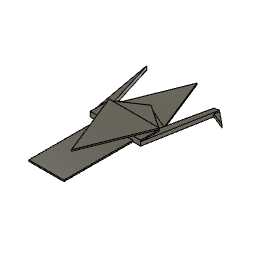
OrigamiBookmark v4 (Autodesk Fusion 360 design; units mm, degrees)
Autodesk Fusion 360 part; units mm, degrees
note: some values were not read from the file. Chosen so that the rebuilt part matches the saved one: which bodies a step acts on. Set by a fixed rule: which sketch regions a step uses.
sketch "Sketch1" plane through (0, 0, 0) normal (0, 0, 1) x (1, 0, 0)
  line L0 (18.6165, 3.413) -> (0.0203, 50.0507)
  line L1 (-20, 0) -> (0, -50)
  line L2 (20, 0) -> (0, -50)
  line L3 (-20, -15) -> (-14, -15)
  line L4 (-20, -15) -> (-20, -0.0774)
  line L5 (-20, -15) -> (-30, 40)
  line L6 (-20, -10) -> (-20, -20) construction
  line L7 (20, -15) -> (14, -15)
  line L8 (20, -15) -> (20, 0)
  line L9 (20, -15) -> (29.6805, 38.2428)
  line L10 (28.9908, 34.4493) -> (40, 30)
  line L11 (29.2258, 38.7285) -> (40, 30)
  line L12 (-17.9674, 1.3624) -> (-30, 40)
  line L13 (29.2258, 38.7285) -> (26.0078, 37.4454)
  line L14 (-18.606, 3.413) -> (18.6165, 3.413) construction
  line L15 (18.1455, 1.2446) -> (26.0078, 37.4454)
  line L16 (29.6805, 38.2428) -> (26.0078, 37.4454)
  line L17 (29.6805, 38.2428) -> (29.7947, 38.2676)
  line L18 (0.0129, 13.4141) -> (-20, 0)
  line L19 (0.0129, 13.4141) -> (20, 0)
  line L20 (0.0129, 13.4141) -> (-17.679, 5.7341)
  line L21 (0, 0) -> (0.219, 1.2047)
  line L22 (0.0203, 50.0507) -> (0.0052, 3.413) construction
  line L23 (0.0129, 13.4141) -> (17.6955, 5.7226)
  line L24 (-18.606, 3.413) -> (0.0203, 50.0507)
  line L25 (-20, 0) -> (-20, -0.0774)
  line L26 (-20, 0) -> (20, 0)
  line L27 (-14, -15) -> (-14, -115)
  line L28 (14, -15) -> (14, -115)
  line L29 (-14, -15) -> (14, -15)
  line L30 (-14, -115) -> (-14, -140)
  line L31 (14, -115) -> (14, -140)
  line L32 (14, -140) -> (-14, -140)
  dimension "d13" = 100
  dimension "d14" = 100
  constraint coincident L1 L3.end
  constraint horizontal L3
  constraint perpendicular L3 L4
  constraint perpendicular L3 L6
  constraint midpoint L3.start L6
  constraint coincident L2 L7.end
  constraint perpendicular L7 L8
  constraint coincident L9 L10.start
  constraint perpendicular L0 L13
  constraint horizontal L14
  constraint coincident L11 L17.end
  constraint parallel L16 L17
  constraint coincident L21.start origin
  constraint parallel L9 L21
  constraint midpoint L14 L22.end
  constraint coincident L0 L23.end
  constraint coincident L19 L15.start
  constraint coincident L0.start L15
  constraint coincident L18 L12.start
  constraint coincident L14.start L12
  constraint parallel L4 L25
  constraint perpendicular L8 L26
  constraint perpendicular L3 L27
  constraint perpendicular L7 L28
  constraint perpendicular L28 L29
  constraint perpendicular L30 L32
  measures "d13" distance of L3.end L27.end
  measures "d14" distance of L7.end L28.end
extrude "Extrude1" add sketch "Sketch1" along normal blind 1 contours L0 L20 L23 L24 makes body 1
extrude "Extrude2" add sketch "Sketch1" along normal blind 2 separate body contours L0 L15 L19 L23 | L11 L13 L16 L17 | L12 L18 L20 L24 makes body 2 at (-5.9806, 9.3969, 0.6667) makes body 2 at (6.0571, 9.3576, 0.6667) makes body 3 at (27.2701, 37.7194, 1.3333)
extrude "Extrude3" add sketch "Sketch1" along normal blind 3 contours L8 L9 L15 L16 L19 | L4 L5 L12 L18 L25 bodies 3 2
extrude "Extrude4" add sketch "Sketch1" along normal blind 2 separate body contours L9 L10 L11 L17 makes body 4
extrude "Extrude5" add sketch "Sketch1" along normal blind 4 contours L18 L19 L26 | L2 L7 L8 | L1 L3 L4 L25 bodies 3 4 1
extrude "Extrude6" add sketch "Sketch1" along normal blind 5 contours L1 L2 L26 L29 | L1 L2 L29 bodies 3
sketch "Sketch2" plane through (0, 0, 0) normal (0, 0, 1) x (1, 0, 0)
sketch "Sketch3" plane through (0, 0, 0) normal (0, 0, 1) x (1, 0, 0)
  line L0 (-14, -15) -> (-14, -115)
  line L1 (-14, -15) -> (14, -15)
  line L2 (14, -15) -> (14, -115)
  line L3 (-14, -115) -> (14, -115)
  line L4 (-14, -115) -> (14, -115)
  line L5 (14, -15) -> (-14, -15)
  line L6 (-14, -115) -> (-14, -15)
  line L7 (-14, -115) -> (-14, -140)
  line L8 (14, -115) -> (14, -140)
  line L9 (14, -140) -> (-14, -140)
  constraint coincident L0.end L3.start
  constraint coincident L2.end L3.end
  constraint coincident L1.end L2.start
  constraint coincident L0.start L1.start
  constraint perpendicular L3 L7
  constraint perpendicular L4 L8
  constraint perpendicular L8 L9
extrude "Extrude7" cut sketch "Sketch3" along normal blind 4 contours L0 L1 L2 L3 L4 L5 L6 bodies 3
extrude "Extrude8" add sketch "Sketch1" along normal blind 1 contours L1 L2 L27 L28 L30 L31 L32 | L1 L2 L29 bodies 3
sketch "Sketch4" plane through (0, 0, 1) normal (0, 0, 1) x (-1, 0, 0)
  line L0 (-14, 140) -> (-14, 15)
  line L1 (-14, 15) -> (14, 15)
  line L2 (14, 15) -> (14, 140)
  line L3 (20, 0) -> (0, 50)
  line L4 (-20, 0) -> (0, 50)
  line L5 (-14, 140) -> (14, 140)
  line L6 (14, 140) -> (-14, 140)
sketch "Sketch6" plane through (0, 0, 1) normal (0, 0, 1) x (-1, 0, 0)
  line L0 (14, 15) -> (14, 140)
  line L1 (14, 140) -> (-14, 140)
  line L2 (-14, 140) -> (-14, 15)
  line L3 (-14, 15) -> (14, 15)
  line L4 (0, -50) -> (0, 140)
  line L5 (0, 140) -> (0, 70)
  line L6 (14, 70) -> (-14, 70)
  constraint midpoint L1 L4.end
  constraint perpendicular L1 L4
  constraint coincident L4 L5.end
  constraint coincident L0 L6.start
  constraint coincident L2 L6.end
  constraint perpendicular L2 L6
extrude "Extrude10" cut sketch "Sketch6" against normal blind 1 contours L0 L1 L4 L5 L6 | L1 L2 L4 L5 L6 bodies 3
sketch "Sketch5" plane through (0, 0, 1) normal (0, 0, 1) x (-1, 0, 0)
  line L0 (14, 115) -> (14, 140)
  line L1 (14, 140) -> (-14, 140)
  line L2 (-14, 140) -> (-14, 115)
  line L3 (-14, 115) -> (14, 115)
